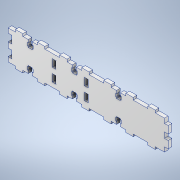
# Autodesk Inventor part: FrontFrame
Saved by Autodesk Inventor 2021 (Build 250183000, 183)
## iProperties
Created: 2021-03-05
Part Number: FrontFrame
Material: Aluminum 6061
Document SubType Name: Modeling
Designer: M3rob
Density: 2.7 g/cm^3
Appearance: Aluminum - Flat
Mass: 1854.16 g
Surface Area: 1368.97 cm^2
Volume: 686.727 cm^3
Author: M3rob
Autodesk Inventor part; units mm, degrees
ref_plane "YZ Plane" through (0, 0, 0) normal (1, 0, 0) x (0, 1, 0)
ref_plane "XZ Plane" through (0, 0, 0) normal (0, 1, 0) x (-1, 0, 0)
ref_plane "XY Plane" through (0, 0, 0) normal (0, 0, 1) x (1, 0, 0)
sketch "Sketch1" plane through (0, 0, 0) normal (0, 0, 1) x (1, 0, 0)
  line L0 (-269.875, 50.8) -> (269.875, 50.8)
  line L1 (269.875, 50.8) -> (269.875, 34.925)
  line L2 (269.875, -50.8) -> (-269.875, -50.8)
  line L3 (-269.875, -50.8) -> (-269.875, -34.925)
  line L4 (0, 50.8) -> (0, -50.8) construction
  line L5 (-269.875, 0) -> (0, 0) construction
  line L6 (-269.875, 34.925) -> (-257.175, 34.925)
  line L7 (-257.175, 34.925) -> (-257.175, 9.525)
  line L8 (-257.175, 9.525) -> (-269.875, 9.525)
  line L9 (-269.875, -9.525) -> (-257.175, -9.525)
  line L10 (-257.175, -9.525) -> (-257.175, -34.925)
  line L11 (-257.175, -34.925) -> (-269.875, -34.925)
  line L12 (-269.875, 34.925) -> (-269.875, 50.8)
  line L13 (-269.875, 9.525) -> (-269.875, 34.925) construction
  line L14 (-269.875, -34.925) -> (-269.875, -9.525) construction
  line L15 (-269.875, -9.525) -> (-269.875, 9.525)
  line L16 (269.875, 34.925) -> (282.575, 34.925)
  line L17 (282.575, 34.925) -> (282.575, 9.525)
  line L18 (282.575, 9.525) -> (269.875, 9.525)
  line L19 (269.875, -9.525) -> (282.575, -9.525)
  line L20 (282.575, -9.525) -> (282.575, -34.925)
  line L21 (282.575, -34.925) -> (269.875, -34.925)
  line L22 (269.875, 9.525) -> (269.875, -9.525)
  line L23 (269.875, 34.925) -> (269.875, 9.525) construction
  line L24 (269.875, -9.525) -> (269.875, -34.925) construction
  line L25 (269.875, -34.925) -> (269.875, -50.8)
  line L26 (-244.475, 58.7375) -> (-219.075, 58.7375)
  line L27 (-219.075, 58.7375) -> (-219.075, 42.8625)
  line L28 (-219.075, 42.8625) -> (-244.475, 42.8625)
  line L29 (-244.475, 42.8625) -> (-244.475, 58.7375)
  line L30 (-244.475, -58.7375) -> (-219.075, -58.7375)
  line L31 (-219.075, -58.7375) -> (-219.075, -42.8625)
  line L32 (-219.075, -42.8625) -> (-244.475, -42.8625)
  line L33 (-244.475, -42.8625) -> (-244.475, -58.7375)
  line L34 (-142.875, 42.8625) -> (-168.275, 42.8625)
  line L35 (-142.875, 58.7375) -> (-142.875, 42.8625)
  line L36 (-168.275, 58.7375) -> (-142.875, 58.7375)
  line L37 (-168.275, 42.8625) -> (-168.275, 58.7375)
  line L38 (-142.875, -42.8625) -> (-168.275, -42.8625)
  line L39 (-142.875, -58.7375) -> (-142.875, -42.8625)
  line L40 (-168.275, -42.8625) -> (-168.275, -58.7375)
  line L41 (-168.275, -58.7375) -> (-142.875, -58.7375)
  line L42 (-66.675, 42.8625) -> (-92.075, 42.8625)
  line L43 (-66.675, 58.7375) -> (-66.675, 42.8625)
  line L44 (-92.075, 58.7375) -> (-66.675, 58.7375)
  line L45 (-92.075, 42.8625) -> (-92.075, 58.7375)
  line L46 (-66.675, -42.8625) -> (-92.075, -42.8625)
  line L47 (-66.675, -58.7375) -> (-66.675, -42.8625)
  line L48 (-92.075, -42.8625) -> (-92.075, -58.7375)
  line L49 (-92.075, -58.7375) -> (-66.675, -58.7375)
  line L50 (9.525, 42.8625) -> (-15.875, 42.8625)
  line L51 (9.525, 58.7375) -> (9.525, 42.8625)
  line L52 (-15.875, 58.7375) -> (9.525, 58.7375)
  line L53 (-15.875, 42.8625) -> (-15.875, 58.7375)
  line L54 (9.525, -42.8625) -> (-15.875, -42.8625)
  line L55 (9.525, -58.7375) -> (9.525, -42.8625)
  line L56 (-15.875, -42.8625) -> (-15.875, -58.7375)
  line L57 (-15.875, -58.7375) -> (9.525, -58.7375)
  line L58 (85.725, 42.8625) -> (60.325, 42.8625)
  line L59 (85.725, 58.7375) -> (85.725, 42.8625)
  line L60 (60.325, 58.7375) -> (85.725, 58.7375)
  line L61 (60.325, 42.8625) -> (60.325, 58.7375)
  line L62 (85.725, -42.8625) -> (60.325, -42.8625)
  line L63 (85.725, -58.7375) -> (85.725, -42.8625)
  line L64 (60.325, -42.8625) -> (60.325, -58.7375)
  line L65 (60.325, -58.7375) -> (85.725, -58.7375)
  line L66 (161.925, 42.8625) -> (136.525, 42.8625)
  line L67 (161.925, 58.7375) -> (161.925, 42.8625)
  line L68 (136.525, 58.7375) -> (161.925, 58.7375)
  line L69 (136.525, 42.8625) -> (136.525, 58.7375)
  line L70 (161.925, -42.8625) -> (136.525, -42.8625)
  line L71 (161.925, -58.7375) -> (161.925, -42.8625)
  line L72 (136.525, -42.8625) -> (136.525, -58.7375)
  line L73 (136.525, -58.7375) -> (161.925, -58.7375)
  line L74 (238.125, 42.8625) -> (212.725, 42.8625)
  line L75 (238.125, 58.7375) -> (238.125, 42.8625)
  line L76 (212.725, 58.7375) -> (238.125, 58.7375)
  line L77 (212.725, 42.8625) -> (212.725, 58.7375)
  line L78 (238.125, -42.8625) -> (212.725, -42.8625)
  line L79 (238.125, -58.7375) -> (238.125, -42.8625)
  line L80 (212.725, -42.8625) -> (212.725, -58.7375)
  line L81 (212.725, -58.7375) -> (238.125, -58.7375)
  line L82 (-6.35, 34.925) -> (6.35, 34.925)
  line L83 (6.35, 34.925) -> (6.35, 9.525)
  line L84 (6.35, 9.525) -> (-6.35, 9.525)
  line L85 (-6.35, 9.525) -> (-6.35, 34.925)
  line L86 (-6.35, -9.525) -> (6.35, -9.525)
  line L87 (6.35, -9.525) -> (6.35, -34.925)
  line L88 (6.35, -34.925) -> (-6.35, -34.925)
  line L89 (-6.35, -34.925) -> (-6.35, -9.525)
  line L90 (-200.4187, 50.8) -> (-200.4187, 41.275)
  line L91 (-200.4187, 41.275) -> (-203.2, 41.275)
  line L92 (-203.2, 41.275) -> (-203.2, 30.1625)
  line L93 (-203.2, 30.1625) -> (-200.4187, 30.1625)
  line L94 (-200.4187, 30.1625) -> (-200.4187, 26.9875)
  line L95 (-200.4187, 26.9875) -> (-186.9313, 26.9875)
  line L96 (-186.9313, 26.9875) -> (-186.9313, 30.1625)
  line L97 (-186.9313, 30.1625) -> (-184.15, 30.1625)
  line L98 (-184.15, 30.1625) -> (-184.15, 41.275)
  line L99 (-184.15, 41.275) -> (-186.9313, 41.275)
  line L100 (-186.9313, 50.8) -> (-186.9313, 41.275)
  line L101 (-193.675, 50.8) -> (-193.675, 26.9875) construction
  line L102 (-200.4187, 50.8) -> (-186.9313, 50.8)
  line L103 (-200.4187, -50.8) -> (-200.4187, -41.275)
  line L104 (-200.4187, -41.275) -> (-203.2, -41.275)
  line L105 (-203.2, -41.275) -> (-203.2, -30.1625)
  line L106 (-203.2, -30.1625) -> (-200.4187, -30.1625)
  line L107 (-200.4187, -30.1625) -> (-200.4187, -26.9875)
  line L108 (-200.4187, -26.9875) -> (-186.9313, -26.9875)
  line L109 (-186.9313, -26.9875) -> (-186.9313, -30.1625)
  line L110 (-186.9313, -30.1625) -> (-184.15, -30.1625)
  line L111 (-184.15, -30.1625) -> (-184.15, -41.275)
  line L112 (-184.15, -41.275) -> (-186.9313, -41.275)
  line L113 (-186.9313, -50.8) -> (-186.9313, -41.275)
  line L114 (-193.675, -50.8) -> (-193.675, -26.9875) construction
  line L115 (-200.4187, -50.8) -> (-186.9313, -50.8)
  line L116 (-48.0187, 41.275) -> (-50.8, 41.275)
  line L117 (-48.0187, 50.8) -> (-48.0187, 41.275)
  line L118 (-50.8, 41.275) -> (-50.8, 30.1625)
  line L119 (-50.8, 30.1625) -> (-48.0187, 30.1625)
  line L120 (-48.0187, 30.1625) -> (-48.0187, 26.9875)
  line L121 (-48.0187, 50.8) -> (-34.5313, 50.8)
  line L122 (-41.275, 50.8) -> (-41.275, 26.9875) construction
  line L123 (-34.5313, 50.8) -> (-34.5313, 41.275)
  line L124 (-31.75, 41.275) -> (-34.5313, 41.275)
  line L125 (-48.0187, 26.9875) -> (-34.5313, 26.9875)
  line L126 (-34.5313, 26.9875) -> (-34.5313, 30.1625)
  line L127 (-31.75, 30.1625) -> (-31.75, 41.275)
  line L128 (-34.5313, 30.1625) -> (-31.75, 30.1625)
  line L129 (-31.75, -41.275) -> (-34.5313, -41.275)
  line L130 (-31.75, -30.1625) -> (-31.75, -41.275)
  line L131 (-34.5313, -30.1625) -> (-31.75, -30.1625)
  line L132 (-48.0187, -30.1625) -> (-48.0187, -26.9875)
  line L133 (-48.0187, -26.9875) -> (-34.5313, -26.9875)
  line L134 (-34.5313, -26.9875) -> (-34.5313, -30.1625)
  line L135 (-41.275, -50.8) -> (-41.275, -26.9875) construction
  line L136 (-34.5313, -50.8) -> (-34.5313, -41.275)
  line L137 (-48.0187, -50.8) -> (-34.5313, -50.8)
  line L138 (-48.0187, -50.8) -> (-48.0187, -41.275)
  line L139 (-48.0187, -41.275) -> (-50.8, -41.275)
  line L140 (-50.8, -30.1625) -> (-48.0187, -30.1625)
  line L141 (-50.8, -41.275) -> (-50.8, -30.1625)
  line L142 (104.3813, 41.275) -> (101.6, 41.275)
  line L143 (104.3813, 50.8) -> (104.3813, 41.275)
  line L144 (101.6, 41.275) -> (101.6, 30.1625)
  line L145 (101.6, 30.1625) -> (104.3813, 30.1625)
  line L146 (104.3813, 30.1625) -> (104.3813, 26.9875)
  line L147 (104.3813, 50.8) -> (117.8687, 50.8)
  line L148 (111.125, 50.8) -> (111.125, 26.9875) construction
  line L149 (117.8687, 50.8) -> (117.8687, 41.275)
  line L150 (120.65, 41.275) -> (117.8687, 41.275)
  line L151 (104.3813, 26.9875) -> (117.8687, 26.9875)
  line L152 (117.8687, 26.9875) -> (117.8687, 30.1625)
  line L153 (120.65, 30.1625) -> (120.65, 41.275)
  line L154 (117.8687, 30.1625) -> (120.65, 30.1625)
  line L155 (120.65, -41.275) -> (117.8687, -41.275)
  line L156 (120.65, -30.1625) -> (120.65, -41.275)
  line L157 (117.8687, -30.1625) -> (120.65, -30.1625)
  line L158 (104.3813, -30.1625) -> (104.3813, -26.9875)
  line L159 (104.3813, -26.9875) -> (117.8687, -26.9875)
  line L160 (117.8687, -26.9875) -> (117.8687, -30.1625)
  line L161 (111.125, -50.8) -> (111.125, -26.9875) construction
  line L162 (117.8687, -50.8) -> (117.8687, -41.275)
  line L163 (104.3813, -50.8) -> (117.8687, -50.8)
  line L164 (104.3813, -50.8) -> (104.3813, -41.275)
  line L165 (104.3813, -41.275) -> (101.6, -41.275)
  line L166 (101.6, -30.1625) -> (104.3813, -30.1625)
  line L167 (101.6, -41.275) -> (101.6, -30.1625)
  line L168 (-104.775, 9.525) -> (-117.475, 9.525)
  line L169 (-117.475, 34.925) -> (-104.775, 34.925)
  line L170 (-104.775, 34.925) -> (-104.775, 9.525)
  line L171 (-117.475, 9.525) -> (-117.475, 34.925)
  line L172 (-104.775, -34.925) -> (-117.475, -34.925)
  line L173 (-117.475, -9.525) -> (-104.775, -9.525)
  line L174 (-104.775, -9.525) -> (-104.775, -34.925)
  line L175 (-117.475, -34.925) -> (-117.475, -9.525)
  point P0 (-219.075, 50.8)
  point P1 (-219.075, -50.8)
  point P2 (-142.875, 50.8)
  point P3 (-142.875, -50.8)
  point P4 (-66.675, 50.8)
  point P5 (-66.675, -50.8)
  point P6 (9.525, 50.8)
  point P7 (9.525, -50.8)
  point P8 (85.725, 50.8)
  point P9 (85.725, -50.8)
  point P10 (161.925, 50.8)
  point P11 (161.925, -50.8)
  point P12 (238.125, 50.8)
  point P13 (238.125, -50.8)
  point P14 (238.125, -50.8)
  point P15 (238.125, 50.8)
  point P16 (212.725, 50.8)
  point P17 (161.925, 50.8)
  point P18 (136.525, 50.8)
  point P19 (85.725, 50.8)
  point P20 (60.325, 50.8)
  point P21 (9.525, 50.8)
  point P22 (-15.875, 50.8)
  point P23 (-66.675, 50.8)
  point P24 (-92.075, 50.8)
  point P25 (-142.875, 50.8)
  point P26 (-168.275, 50.8)
  point P27 (-244.475, 50.8)
  point P28 (-244.475, -50.8)
  point P29 (-219.075, -50.8)
  point P30 (-168.275, -50.8)
  point P31 (-142.875, -50.8)
  point P32 (-92.075, -50.8)
  point P33 (-66.675, -50.8)
  point P34 (-15.875, -50.8)
  point P35 (9.525, -50.8)
  point P36 (60.325, -50.8)
  point P37 (85.725, -50.8)
  point P38 (136.525, -50.8)
  point P39 (161.925, -50.8)
  point P40 (212.725, -50.8)
  point P41 (0, 9.525)
  point P42 (0, -9.525)
  point P43 (117.8687, 50.8)
  point P44 (104.3813, 50.8)
  point P45 (-34.5313, 50.8)
  point P46 (-48.0187, 50.8)
  point P47 (-48.0187, -50.8)
  point P48 (-34.5313, -50.8)
  point P49 (-111.125, 9.525)
  point P50 (-111.125, -9.525)
  dimension "d0" = 539.75
  dimension "d1" = 101.6
  dimension "d2" = 269.875
  dimension "d3" = 19.05
  dimension "d4" = 25.4
  dimension "d5" = 25.4
  dimension "d6" = 12.7
  dimension "d7" = 25.4
  dimension "d8" = 7.9375
  dimension "d9" = 25.4
  dimension "d12" = 76.2
  dimension "d19" = 9.525
  dimension "d20" = 11.1125
  dimension "d21" = 3.175
  dimension "d22" = 19.05
  dimension "d23" = 13.4874
  dimension "d24" = 25.4
  dimension "d30" = 152.4
  dimension "d34" = 111.125
  constraints: 348 end point, 63 horizontal alignment, 58 point on line, 56 parallel, 33 perpendicular, 24 collinear, 21 symmetric about line, 9 horizontal, 7 vertical, 6 midpoint, 5 equal length, 1 coincident, 1 vertical alignment, 142 other
  measures "d0" distance of L12.end L1.start
  measures "d1" distance of L1.start L25.end
  measures "d2" distance of L5.start L5.end
  measures "d3" distance between parallel lines of L9 L8
  measures "d4" distance of L6.end L7.end
  measures "d5" distance of L9.end L10.end
  measures "d6" distance of L9.start L9.end
  measures "d7" distance of L26.start L26.end
  measures "d9" horizontal distance of L12.end L28.end
  measures "d12" distance of L27.end L34.start
  measures "d19" distance of L100.start L99.end
  measures "d20" distance of L97.end L98.end
  measures "d21" distance of L95.end L96.end
  measures "d22" distance between parallel lines of L92 L98
  measures "d23" distance between parallel lines of L100 L90
  measures "d24" distance from line of L27 L101.start
  measures "d30" distance of L91.end L116.end
  measures "d34" distance of L83.end L168.start
extrude "Extrusion1" add sketch "Sketch1" along normal mid plane 12.7 contours L90 L91 L92 L93 L94 L95 L96 L97 L98 L99 L100 L0 L37 L34 L35 L45 L42 L43 L117 L116 L118 L119 L120 L125 L126 L128 L127 L124 L123 L53 L50 L51 L61 L58 L59 L143 L142 L144 L145 L146 L151 L152 L154 L153 L150 L149 L69 L66 L67 L77 L74 L75 L1 L16 L17 L18 L22 L19 L20 L21 L25 L2 L79 L78 L80 L71 L70 L72 L162 L155 L156 L157 L160 L159 L158 L166 L167 L165 L164 L63 L62 L64 L55 L54 L56 L136 L129 L130 L131 L134 L133 L132 L140 L141 L139 L138 L47 L46 L48 L39 L38 L40 L113 L112 L111 L110 L109 L108 L107 L106 L105 L104 L103 L31 L32 L33 L3 L11 L10 L9 L15 L8 L7 L6 L12 L29 L28 L27 | L27 L28 L29 L0 | L0 L29 L26 L27 | L37 L36 L35 L0 | L0 L35 L34 L37 | L45 L44 L43 L0 | L0 L43 L42 L45 | L53 L52 L51 L0 | L0 L51 L50 L53 | L61 L60 L59 L0 | L0 L59 L58 L61 | L33 L32 L31 L2 | L2 L31 L30 L33 | L69 L68 L67 L0 | L0 L67 L66 L69 | L77 L76 L75 L0 | L0 L75 L74 L77 | L40 L38 L39 L2 | L2 L39 L41 L40 | L48 L46 L47 L2 | L2 L47 L49 L48 | L56 L54 L55 L2 | L2 L55 L57 L56 | L64 L62 L63 L2 | L2 L63 L65 L64 | L79 L81 L80 L2 | L2 L80 L78 L79 | L72 L70 L71 L2 | L2 L71 L73 L72
equation "\"d2\" = 0.5 * d0"
body "Solid1"
